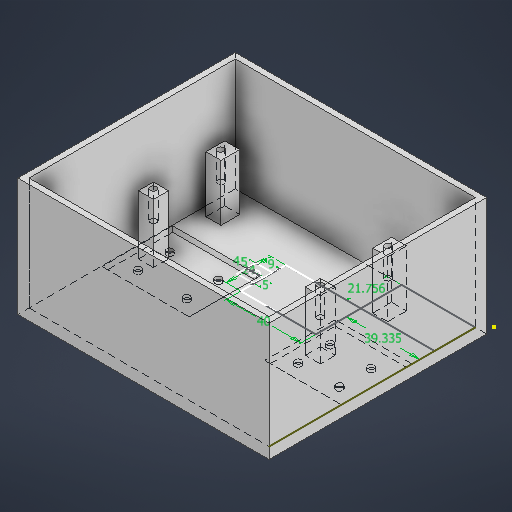
# Autodesk Inventor part: BOTTOM
Saved by Autodesk Inventor 2026.1 (Build 301233020, 233B)
## iProperties
Created: 2026-07-07
Part Number: BOTTOM
Material: Generic
Document SubType Name: Modeling
Designer: pleased
Density: 1 g/cm^3
Appearance: Default
Author: pleased
Autodesk Inventor part; units mm, degrees
ref_plane "YZ Plane" through (0, 0, 0) normal (1, 0, 0) x (0, 1, 0)
ref_plane "XZ Plane" through (0, 0, 0) normal (0, 1, 0) x (-1, 0, 0)
ref_plane "XY Plane" through (0, 0, 0) normal (0, 0, 1) x (1, 0, 0)
sketch "Sketch1" plane through (0, 0, 0) normal (0, 1, 0) x (-1, 0, 0)
  line L0 (0, 120) -> (138, 120)
  line L1 (138, 120) -> (138, 0)
  line L2 (138, 0) -> (0, 0)
  line L3 (0, 0) -> (0, 120)
  point P0 (0, 0)
  dimension "d0" = 138
  dimension "d1" = 120
  constraints: 8 end point, 2 parallel, 1 horizontal, 1 perpendicular
  measures "d0" distance of L1.end L2.end
  measures "d1" distance of L0.end L1.end
extrude "Extrusion1" add sketch "Sketch1" along normal blind 3
sketch "Sketch2" plane through (0, 3, 0) normal (0, 1, 0) x (1, 0, 0)
  circle A0 centre (-123.5, -66.5) radius 1.75
  circle A1 centre (-123.5, -49.5) radius 1.75
  circle A2 centre (-97.5, -66.5) radius 1.75
  circle A3 centre (-97.5, -49.5) radius 1.75
  circle A4 centre (-38, -66.5) radius 1.75
  circle A5 centre (-38, -49.5) radius 1.75
  circle A6 centre (-16, -66.5) radius 1.75
  circle A7 centre (-16, -49.5) radius 1.75
  point P0 (0, 0)
  dimension "d5" = 3.5
  dimension "d6" = 3.5
  dimension "d7" = 3.5
  dimension "d8" = 3.5
  dimension "d9" = 3.5
  dimension "d10" = 3.5
  dimension "d11" = 3.5
  dimension "d12" = 3.5
  constraints: 8 centre point, 8 coincident
  measures "d5" diameter of A0
  measures "d6" diameter of A1
  measures "d7" diameter of A2
  measures "d8" diameter of A3
  measures "d9" diameter of A4
  measures "d10" diameter of A5
  measures "d11" diameter of A6
  measures "d12" diameter of A7
extrude "Extrusion2" cut sketch "Sketch2" against normal blind 3
sketch "Sketch3" plane through (0, 3, 0) normal (0, 1, 0) x (1, 0, 0)
  line L0 (-131.1985, -74.9193) -> (-87.7046, -74.9193)
  line L1 (-87.7046, -74.9193) -> (-87.7046, -40.2677)
  line L2 (-87.7046, -40.2677) -> (-131.1985, -40.2677)
  line L3 (-131.1985, -40.2677) -> (-131.1985, -74.9193)
  line L4 (-44.4498, -74.9193) -> (-6.6914, -74.9193)
  line L5 (-6.6914, -74.9193) -> (-6.6914, -40.2677)
  line L6 (-6.6914, -40.2677) -> (-44.4498, -40.2677)
  line L7 (-44.4498, -40.2677) -> (-44.4498, -74.9193)
  point P0 (0, 0)
  constraints: 16 end point, 4 parallel, 2 horizontal, 2 perpendicular, 2 point on line
extrude "Extrusion3" cut sketch "Sketch3" against normal blind 1.5
chamfer "Chamfer1" distance 1.5 angle 45 8 edges at (-131.1985, 3, 57.5935) (-109.4515, 3, 40.2677) (-109.4515, 3, 74.9193) (-87.7046, 3, 57.5935) (-44.4498, 3, 57.5935) (-25.5706, 3, 40.2677) (-6.6914, 3, 57.5935) (-25.5706, 3, 74.9193)
sketch "Sketch4" plane through (0, 3, 0) normal (0, 1, 0) x (1, 0, 0)
  line L0 (0, 0) -> (-138, 0) projected
  line L1 (-138, -120) -> (0, -120)
  line L2 (0, -120) -> (0, 0)
  line L3 (0, 0) -> (-138, 0)
  line L4 (-138, 0) -> (-138, -120)
  line L5 (-133, -115) -> (-5, -115)
  line L6 (-5, -115) -> (-5, -5)
  line L7 (-5, -5) -> (-133, -5)
  line L8 (-133, -5) -> (-133, -115)
  line L9 (-136, -118) -> (-2, -118)
  line L10 (-2, -118) -> (-2, -2)
  line L11 (-2, -2) -> (-136, -2)
  line L12 (-136, -2) -> (-136, -118)
  dimension "d20" = 5
  dimension "d21" = 3
  constraints: 24 end point, 6 parallel, 3 perpendicular, 1 horizontal, 6 other
  measures "d20" distance between parallel lines of L4 L8
  measures "d21" distance between parallel lines of L8 L12
extrude "Extrusion4" add sketch "Sketch4" along normal blind 60 contours L12 L11 L10 L9
move faces "Move1" translate (0, 0, -2) faces at (-92, 1, 120)
move faces "Move2" translate (-2, 0, 0) faces at (0, 1, 78.6667)
move faces "Move3" translate (0, 0, 2) faces at (-47.3333, 1, 0)
move faces "Move4" translate (2, 0, 0) faces at (-138, 1, 40.6667)
sketch "Sketch5" plane through (0, 3, 0) normal (0, 1, 0) x (1, 0, 0)
  line L0 (-128, -59.6934) -> (-33, -59.6934)
  line L1 (-33, -59.6934) -> (-33, -17.6934)
  line L2 (-33, -17.6934) -> (-128, -17.6934)
  line L3 (-128, -17.6934) -> (-128, -59.6934)
  line L4 (-5, -5) -> (-133, -5) projected
  line L5 (-33, -17.6934) -> (-34, -17.6934)
  line L6 (-33, -18.6934) -> (-33, -17.6934)
  line L7 (-33, -17.6934) -> (-39, -17.6934)
  line L8 (-39, -17.6934) -> (-39, -23.6934)
  line L9 (-39, -23.6934) -> (-33, -23.6934)
  line L10 (-33, -23.6934) -> (-33, -17.6934)
  line L11 (-128, -17.6934) -> (-122, -17.6934)
  line L12 (-122, -17.6934) -> (-122, -23.6934)
  line L13 (-122, -23.6934) -> (-128, -23.6934)
  line L14 (-128, -23.6934) -> (-128, -17.6934)
  line L15 (-128, -59.6934) -> (-122, -59.6934)
  line L16 (-122, -59.6934) -> (-122, -53.6934)
  line L17 (-122, -53.6934) -> (-128, -53.6934)
  line L18 (-128, -53.6934) -> (-128, -59.6934)
  line L19 (-33, -59.6934) -> (-39, -59.6934)
  line L20 (-39, -59.6934) -> (-39, -53.6934)
  line L21 (-39, -53.6934) -> (-33, -53.6934)
  line L22 (-33, -53.6934) -> (-33, -59.6934)
  point P0 (0, 0)
  dimension "d36" = 95
  dimension "d37" = 42
  dimension "d50" = 6
  dimension "d51" = 6
  dimension "d52" = 6
  dimension "d53" = 6
  dimension "d54" = 6
  dimension "d55" = 6
  dimension "d56" = 6
  dimension "d57" = 6
  constraints: 44 end point, 10 parallel, 6 horizontal, 5 perpendicular
  measures "d36" distance of L2.end L1.end
  measures "d37" distance of L1.end L0.end
  measures "d50" distance of L9.end L8.end
  measures "d51" distance of L8.end L7.end
  measures "d52" distance of L12.end L13.end
  measures "d53" distance of L11.end L12.end
  measures "d54" distance of L17.end L16.end
  measures "d55" distance of L16.end L15.end
  measures "d56" distance of L20.end L21.end
  measures "d57" distance of L19.end L20.end
extrude "Extrusion5" add sketch "Sketch5" along normal blind 30 and the other way blind 3 contours L3 L17 L16 L0 | L20 L21 L1 L0 | L3 L2 L12 L13 | L9 L8 L2 L1
sketch "Sketch6" plane through (0, 33, 0) normal (0, 1, 0) x (1, 0, 0)
  line L0 (-39, -23.6934) -> (-39, -17.6934) projected
  line L1 (-33, -23.6934) -> (-39, -23.6934) projected
  line L2 (-39, -17.6934) -> (-33, -23.6934)
  line L3 (-39, -53.6934) -> (-33, -53.6934) projected
  line L4 (-33, -53.6934) -> (-33, -59.6934) projected
  line L5 (-39, -53.6934) -> (-33, -59.6934)
  line L6 (-128, -53.6934) -> (-128, -59.6934) projected
  line L7 (-128, -59.6934) -> (-122, -59.6934) projected
  line L8 (-128, -53.6934) -> (-122, -59.6934)
  line L9 (-128, -17.6934) -> (-128, -23.6934) projected
  line L10 (-128, -17.6934) -> (-122, -23.6934)
  circle A0 centre (-125, -20.6934) radius 1.75
  circle A1 centre (-125, -56.6934) radius 1.75
  circle A2 centre (-36, -56.6934) radius 1.75
  circle A3 centre (-36, -20.6934) radius 1.75
  point P0 (0, 0)
  dimension "d62" = 3.5
  dimension "d63" = 3.5
  dimension "d64" = 3.5
  dimension "d65" = 3.5
  constraints: 8 end point, 4 centre point, 4 midpoint
  measures "d62" diameter of A0
  measures "d63" diameter of A1
  measures "d64" diameter of A2
  measures "d65" diameter of A3
extrude "Extrusion6" cut sketch "Sketch6" against normal blind 15 contours A3 L2 | L2 A3 | A2 L5 | L5 A2 | A1 L8 | L8 A1 | A0 L10 | L10 A0
move faces "Move5" translate (2, 0, 0) faces at (-122, 12, 57.6934) (-122, 13, 21.6934) (-33, 13, 21.6934) (-33, 12, 57.6934)
move faces "Move6" translate (0, 0, 2) faces at (-33.6667, 23, 23.6934) (-36.3333, 22.5, 59.6934) (-125.3333, 12, 59.6934) (-122.6667, 23, 23.6934)
move faces "Move7" translate (0, 0, -2) faces at (-33.6667, 13, 17.6934) (-122.6667, 13, 17.6934)
sketch "Sketch7" plane through (0, 3, 0) normal (0, 1, 0) x (1, 0, 0)
  line L0 (-5, -115) -> (-5, -5) projected
  line L1 (-5, -5) -> (-44.335, -5)
  line L2 (-44.335, -5) -> (-44.335, -26.7557)
  line L3 (-44.335, -26.7557) -> (-5, -26.7557)
  line L4 (-5, -26.7557) -> (-5, -5)
  line L5 (-44.335, -26.7557) -> (-84.335, -26.7557)
  line L6 (-84.335, -26.7557) -> (-84.335, -50.7557)
  line L7 (-84.335, -50.7557) -> (-44.335, -50.7557)
  line L8 (-44.335, -50.7557) -> (-44.335, -26.7557)
  line L9 (-84.335, -38.7557) -> (-93.335, -38.7557)
  line L10 (-93.335, -38.7557) -> (-93.335, -33.7557)
  line L11 (-93.335, -33.7557) -> (-84.335, -33.7557)
  line L12 (-84.335, -33.7557) -> (-84.335, -38.7557)
  line L13 (-93.335, -38.7557) -> (-84.335, -38.7557)
  line L14 (-84.335, -38.7557) -> (-84.335, -43.7557)
  line L15 (-84.335, -43.7557) -> (-93.335, -43.7557)
  line L16 (-93.335, -43.7557) -> (-93.335, -38.7557)
  circle A0 centre (-88.835, -38.7557) radius 2
  point P0 (0, 0)
  dimension "d77" = 39.335
  dimension "d78" = 21.7557
  dimension "d79" = 40
  dimension "d80" = 24
  dimension "d81" = 9
  dimension "d82" = 5
  dimension "d83" = 5
  dimension "d84" = 4
  constraints: 32 end point, 8 parallel, 4 horizontal, 4 perpendicular, 2 midpoint, 1 centre point, 1 point on line
  measures "d77" distance of L3.end L2.end
  measures "d78" distance of L2.end L1.end
  measures "d79" distance of L7.end L6.end
  measures "d80" distance of L6.end L5.end
  measures "d81" distance of L10.end L11.end
  measures "d82" distance of L9.end L10.end
  measures "d83" distance of L13.end L14.end
  measures "d84" diameter of A0
body "Solid1"
